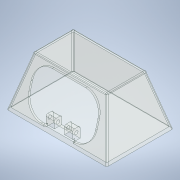
# Autodesk Inventor part: корпус башни
Saved by Autodesk Inventor 2020.1 (Build 241239000, 239)
## iProperties
Created: 2022-03-22
Part Number: корпус башни
Material: Стекло
Document SubType Name: Modeling
Designer: User
Density: 2.18 g/cm^3
Appearance: Бесцветный
Author: User
Autodesk Inventor part; units mm, degrees
ref_plane "YZ Plane" through (0, 0, 0) normal (1, 0, 0) x (0, 1, 0)
ref_plane "XZ Plane" through (0, 0, 0) normal (0, 1, 0) x (-1, 0, 0)
sketch "Эскиз1" plane through (0, 0, 0) normal (0, 0, 1) x (1, 0, 0)
  line L0 (-60, 0) -> (-43.923, 60)
  line L1 (-43.923, 60) -> (43.923, 60)
  line L2 (43.923, 60) -> (60, 0)
  line L3 (60, 0) -> (-60, 0)
  line L4 (0, 0) -> (0, 60)
  dimension "d0" = 120
  dimension "d1" = 75
  dimension "d2" = 60
  constraints: 10 end point, 1 horizontal, 1 midpoint, 1 parallel, 1 perpendicular, 1 other
  measures "d0" distance of L2.end L0.start
  measures "d1" angle of L2 L3
  measures "d2" distance between parallel lines of L3 L1
extrude "Выдавливание1" add sketch "Эскиз1" along normal blind 120
sketch "Эскиз2" plane through (0, 0, 0) normal (1, 0, 0) x (0, 1, 0)
  line L0 (60, 120) -> (0, 120) projected
  line L1 (0, 120) -> (60, 103.923)
  line L2 (60, 0) -> (60, 120) projected
  line L3 (60, 103.923) -> (60, 16.077)
  line L4 (0, 0) -> (0, 120) projected
  line L5 (60, 16.077) -> (0, 0)
  line L6 (0, 0) -> (0, 120)
  line L7 (60, 60) -> (0, 60)
  line L8 (60, 56.077) -> (0, 40)
  point P0 (60, 16.077)
  point P1 (60, 56.077)
  dimension "d5" = 75
  dimension "d36" = 80
  dimension "d37" = 75
  constraints: 12 end point, 3 point on line, 2 midpoint, 1 collinear, 1 perpendicular, 1 vertical, 1 other
  measures "d5" angle of L5 L4
  measures "d36" distance of L8.end L0.end
  measures "d37" angle of L4 L8
extrude "Выдавливание2" cut sketch "Эскиз2" along normal mid plane 120 contours L1 L2 L7 L4 | L7 L2 L8 L4 keep common part
shell "Оболочка1" thickness 2 removed faces 1 at (-20, 0, 66.6667)
ref_plane "РабПлоскость1" through (0, 0, 120) normal (0, 0, 1) x (1, 0, 0)
sketch "Эскиз4" plane through (0, 0, 120) normal (0, 0, 1) x (1, 0, 0)
  circle A0 centre (-20, 35) radius 20
  circle A1 centre (20, 35) radius 20
  circle A2 centre (-20, 25) radius 20
  circle A3 centre (20, 25) radius 20
  line L0 (0, 0) -> (0, 60)
  line L1 (43.923, 60) -> (-43.923, 60) projected
  line L2 (-20, 5) -> (20, 5)
  line L3 (-40, 25) -> (-40, 35)
  line L4 (40, 25) -> (40, 35)
  line L5 (-20, 55) -> (20, 55)
  line L6 (-60, 0) -> (60, 0) projected
  line L7 (-20, 25) -> (-20, 5)
  dimension "d13" = 40
  dimension "d14" = 40
  dimension "d15" = 40
  dimension "d16" = 40
  dimension "d26" = 5
  dimension "d27" = 0
  dimension "d42" = 5
  constraints: 12 end point, 10 tangent, 9 point on circle, 4 centre point, 3 parallel, 1 midpoint, 1 vertical
  measures "d13" diameter of A0
  measures "d14" diameter of A1
  measures "d15" diameter of A2
  measures "d16" diameter of A3
  measures "d26" distance from line of L6 L2.end
  measures "d27" distance of L7.end L2.start
  measures "d42" distance from line of L1 L5.start
extrude "Выдавливание3" cut sketch "Эскиз4" against normal blind 40
sketch "Эскиз5" plane through (-60, 0, 0) normal (0, -1, 0) x (1, 0, 0)
  line L0 (2.0706, 117.9294) -> (117.9294, 117.9294) projected
  line L1 (76, 117.9294) -> (44, 117.9294)
  line L2 (44, 117.9294) -> (44, 107.9294)
  line L3 (44, 107.9294) -> (76, 107.9294)
  line L4 (76, 107.9294) -> (76, 117.9294)
  point P0 (60, 0)
  point P1 (44, 117.9294)
  point P2 (60, 117.9294)
  point P3 (60, 117.9294)
  dimension "d21" = 10
  dimension "d22" = 32
  dimension "d38" = 0
  constraints: 8 end point, 2 midpoint, 2 parallel, 1 horizontal, 1 perpendicular, 1 point on line
  measures "d21" distance of L3.end L1.start
  measures "d22" distance of L2.end L3.end
  measures "d38" distance of point (60, 117.929) point (60, 117.929)
extrude "Выдавливание4" add sketch "Эскиз5" against normal blind 5
sketch "Эскиз6" plane through (-20, 5, 118.6603) normal (0, 1, 0) x (1, 0, 0)
  line L0 (36, 10.7308) -> (4, 10.7308) projected
  line L1 (4, 10.7308) -> (14, 10.7308)
  line L2 (14, 10.7308) -> (14, 2.0706)
  line L3 (14, 2.0706) -> (4, 2.0706)
  line L4 (4, 2.0706) -> (4, 10.7308)
  line L5 (36, 10.7308) -> (26, 10.7308)
  line L6 (26, 10.7308) -> (26, 2.0706)
  line L7 (26, 2.0706) -> (36, 2.0706)
  line L8 (36, 2.0706) -> (36, 10.7308)
  point P0 (20, 118.6603)
  dimension "d28" = 10
  dimension "d29" = 10
  constraints: 16 end point, 4 parallel, 2 horizontal, 2 perpendicular, 1 point on line
  measures "d28" distance of L2.end L3.end
  measures "d29" distance of L7.end L6.end
extrude "Выдавливание5" add sketch "Эскиз6" along normal blind 10
sketch "Эскиз7" plane through (16, 0, 117.9294) normal (1, 0, 0) x (0, 0, -1)
  line L0 (1.3397, 15) -> (10, 15) projected
  line L1 (10, 5) -> (10, 15) projected
  circle A0 centre (5.6699, 10) radius 2
  point P0 (117.9294, 0)
  point P1 (5.6699, 15)
  point P2 (10, 10)
  dimension "d32" = 4
  constraints: 2 midpoint, 1 centre point
  measures "d32" diameter of A0
extrude "Выдавливание6" cut sketch "Эскиз7" against normal blind 40
fillet "Сопряжение1" radius 2 6 edges at (11, 15, 107.9294) (11, 15, 116.5897) (-11, 15, 107.9294) (-11, 15, 116.5897) (16, 2.5, 117.2596) (-16, 2.5, 117.2596)
sketch "Эскиз8" plane through (-60, 0, 40) normal (0, -1, 0) x (1, 0, 0)
  line L0 (117.9294, 77.9294) -> (117.9294, 2.0706) projected
  line L1 (2.0706, 2.0706) -> (17.6116, 17.6116) projected
  line L2 (117.9294, 77.9294) -> (2.0706, 77.9294)
  line L3 (2.0706, 77.9294) -> (2.0706, 2.0706)
  line L4 (2.0706, 2.0706) -> (117.9294, 2.0706)
  line L5 (117.9294, 2.0706) -> (117.9294, 77.9294)
  point P0 (60, -40)
  constraints: 8 end point, 2 parallel, 1 horizontal, 1 perpendicular
extrude "Выдавливание7" add sketch "Эскиз8" against normal blind 2
fillet "Сопряжение2" radius 2 8 edges at (51.9615, 30, 111.9615) (51.9615, 30, 48.0385) (-51.9615, 30, 48.0385) (-51.9615, 30, 111.9615) (0, 60, 56.077) (-43.923, 60, 80) (0, 60, 103.923) (43.923, 60, 80)
equation "\"d19\" = d15"
